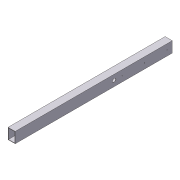
# Autodesk Inventor part: GE-12019-02
Saved by Autodesk Inventor 2012 (Build 160160000, 160)
## iProperties
Created: 2011-06-10
Part Number: GE-12019-02
Document SubType Name: Modeling
Designer: dfoster
Density: 2.71 g/cm^3
Material: Aluminum-6061
Mass: 2165.32 g
Surface Area: 5047.94 cm^2
Volume: 799.011 cm^3
Description: Tube, Cross Brace
Title: Tube, Cross Brace
Author: dfoster
Autodesk Inventor part; units mm, degrees
ref_plane "YZ Plane" through (0, 0, 0) normal (1, 0, 0) x (0, 1, 0)
ref_plane "XZ Plane" through (0, 0, 0) normal (0, 1, 0) x (-1, 0, 0)
ref_plane "XY Plane" through (0, 0, 0) normal (0, 0, 1) x (1, 0, 0)
sketch "Sketch1" plane through (0, 0, 0) normal (0, 0, 1) x (1, 0, 0)
  line L0 (0, 0) -> (50.8, 0)
  line L1 (50.8, 0) -> (50.8, 76.2)
  line L2 (50.8, 76.2) -> (0, 76.2)
  line L3 (0, 76.2) -> (0, 0)
  line L4 (3.175, 73.025) -> (47.625, 73.025)
  line L5 (47.625, 73.025) -> (47.625, 3.175)
  line L6 (47.625, 3.175) -> (3.175, 3.175)
  line L7 (3.175, 3.175) -> (3.175, 73.025)
  dimension "d13" = 3.175
  dimension "d14" = 50.8
  dimension "d15" = 76.2
  dimension "d37" = 3.175
  dimension "d38" = 3.175
  dimension "d39" = 3.175
  constraints: 16 end point, 4 parallel, 2 perpendicular, 1 horizontal
  measures "d13" distance between parallel lines of L4 L2
  measures "d14" distance between parallel lines of L1 L3
  measures "d15" distance between parallel lines of L0 L2
  measures "d37" distance between parallel lines of L7 L3
  measures "d38" distance between parallel lines of L1 L5
  measures "d39" distance between parallel lines of L6 L0
extrude "Extrusion1" add sketch "Sketch1" along normal blind 1117.6
hole "Hole1" at (50.8, 38.1, 412.75) direction (-1, 0, 0) diameter 25.4 end through all
hole "Hole2" at (50.8, 38.1, 38.1) direction (-1, 0, 0) diameter 4.7752 end through all
pattern_linear "Rectangular Pattern1" count 3 spacing 158.75 along (0, 0, 1) of "Hole2"
equation "\"d37\" = d13"
equation "\"d38\" = d13"
equation "\"d39\" = d13"
body "Solid1"
